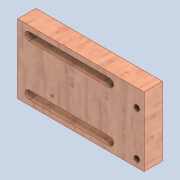
# Autodesk Inventor part: 0005-10-021 suport senzor z
Saved by Autodesk Inventor 2020 (Build 240168000, 168)
## iProperties
Created: 2020-12-18
Part Number: 0005-10-021 suport senzor z
Material: Generic
Document SubType Name: Modeling
Designer: Iulian Bors
Density: 1 g/cm^3
Appearance: White Oak - Natural Medium Gloss
Mass: 9.17008 g
Surface Area: 45.9205 cm^2
Volume: 9.17008 cm^3
Author: Iulian Bors
Subject: 021
Autodesk Inventor part; units mm, degrees
ref_plane "YZ Plane" through (0, 0, 0) normal (1, 0, 0) x (0, 1, 0)
ref_plane "XZ Plane" through (0, 0, 0) normal (0, 1, 0) x (-1, 0, 0)
ref_plane "XY Plane" through (0, 0, 0) normal (0, 0, 1) x (1, 0, 0)
sketch "Sketch1" plane through (0, 0, 0) normal (0, 0, 1) x (1, 0, 0)
  line L0 (-27.5, 15) -> (27.5, 15)
  line L1 (27.5, 15) -> (27.5, -15)
  line L2 (27.5, -15) -> (-27.5, -15)
  line L3 (-27.5, -15) -> (-27.5, 15)
  point P0 (0, 0)
  point P1 (0, 15)
  point P2 (-27.5, 0)
  dimension "d0" = 55
  dimension "d1" = 30
  constraints: 8 end point, 2 midpoint, 2 parallel, 1 horizontal, 1 horizontal alignment, 1 perpendicular, 1 vertical alignment
  measures "d0" distance of L0.start L0.end
  measures "d1" distance of L2.end L0.start
extrude "Extrusion1" add sketch "Sketch1" along normal blind 8
sketch "Sketch5" plane through (0, 0, 8) normal (0, 0, 1) x (1, 0, 0)
  line L0 (12.5, 11) -> (-22.5, 11) construction
  line L1 (12.5, 12.75) -> (-22.5, 12.75)
  line L2 (-22.5, 9.25) -> (12.5, 9.25)
  arc A0 (12.5, 9.25) -> (12.5, 12.75) centre (12.5, 11) ccw
  arc A1 (-22.5, 12.75) -> (-22.5, 9.25) centre (-22.5, 11) ccw
  line L3 (12.5, -11) -> (-22.5, -11) construction
  line L4 (12.5, -9.25) -> (-22.5, -9.25)
  line L5 (-22.5, -12.75) -> (12.5, -12.75)
  arc A2 (12.5, -12.75) -> (12.5, -9.25) centre (12.5, -11) ccw
  arc A3 (-22.5, -9.25) -> (-22.5, -12.75) centre (-22.5, -11) ccw
  line L6 (27.5, 15) -> (-27.5, 15) projected
  line L7 (-27.5, -15) -> (27.5, -15) projected
  line L8 (-27.5, 15) -> (-27.5, -15) projected
  point P0 (0, 0)
  point P1 (-5, 11)
  point P2 (-5, -11)
  dimension "d29" = 3.5
  dimension "d30" = 4
  dimension "d31" = 4
  dimension "d33" = 35
  dimension "d36" = 5
  constraints: 16 end point, 8 point on circle, 8 tangent, 5 parallel, 4 centre point, 2 midpoint, 1 equal radius, 1 horizontal, 1 vertical alignment
  measures "d29" distance between parallel lines of L2 L1
  measures "d30" distance between parallel lines of L0 L6
  measures "d31" distance between parallel lines of L7 L3
  measures "d33" distance of L0.start L0.end
  measures "d36" distance from line of L8 L0.end
extrude "Extrusion5" cut sketch "Sketch5" against normal blind 10
sketch "Sketch6" plane through (0, 0, 8) normal (0, 0, 1) x (1, 0, 0)
  circle A0 centre (24.3725, -11.7625) radius 1.7875
  circle A1 centre (24.3725, 7.4125) radius 1.7875
  line L0 (27.5, -15) -> (27.5, 15) projected
  point P0 (0, 0)
  dimension "d44" = 3.1275
  constraints: 2 centre point, 1 vertical alignment
  measures "d44" distance from line of A1.centre L0
hole "Hole1" at (24.3725, 7.4125, 8) at (24.3725, -11.7625, 8) direction (0, 0, -1) diameter 2.459 end through all thread size "M3x0.5" class "6H" standard "ISO Metric profile"
body "Solid1"
